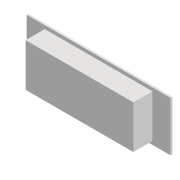
# Autodesk Inventor part: 00_FluidicChip_Vittorio
Saved by Autodesk Inventor 2022 (Build 260153000, 153)
## iProperties
Created: 2021-12-01
Part Number: 00_FluidicChip_Vittorio
Material: Generisch
Document SubType Name: Modeling
Designer: diederichbenedict
Density: 1 g/cm^3
Appearance: Vorgabe
Author: diederichbenedict
Autodesk Inventor part; units mm, degrees
ref_plane "YZ Plane" through (0, 0, 0) normal (1, 0, 0) x (0, 1, 0)
ref_plane "XZ Plane" through (0, 0, 0) normal (0, 1, 0) x (-1, 0, 0)
ref_plane "XY Plane" through (0, 0, 0) normal (0, 0, 1) x (1, 0, 0)
sketch "Skizze1" plane through (0, 0, 0) normal (0, 0, 1) x (1, 0, 0)
  line L0 (37.5, -13) -> (-37.5, -13)
  line L1 (-37.5, -13) -> (-37.5, 13)
  line L2 (-37.5, 13) -> (37.5, 13)
  line L3 (37.5, 13) -> (37.5, -13)
  line L4 (37.5, -13) -> (-37.5, 13) construction
  line L5 (-37.5, -13) -> (37.5, 13) construction
  point P0 (0, 0)
  dimension "d0" = 75
  dimension "d1" = 26
  constraints: 12 end point, 2 midpoint, 2 parallel, 1 horizontal, 1 perpendicular
  measures "d0" distance of L1.end L2.end
  measures "d1" distance of L0.end L1.end
extrude "Extrusion1" add sketch "Skizze1" along normal blind 1
sketch "Skizze2" plane through (0, 0, 1) normal (0, 0, 1) x (1, 0, 0)
  line L0 (37.5, 13) -> (-37.5, 13) projected
  line L1 (-37.5, 13) -> (-37.5, -13) projected
  line L2 (-37.5, -13) -> (37.5, -13) projected
  line L3 (37.5, -13) -> (37.5, 13) projected
  line L4 (28.1272, -11.233) -> (-28.1272, -11.233)
  line L5 (-28.1272, -11.233) -> (-28.1272, 11.233)
  line L6 (-28.1272, 11.233) -> (28.1272, 11.233)
  line L7 (28.1272, 11.233) -> (28.1272, -11.233)
  line L8 (28.1272, -11.233) -> (-28.1272, 11.233) construction
  line L9 (-28.1272, -11.233) -> (28.1272, 11.233) construction
  point P0 (0, 0)
  constraints: 12 end point, 2 midpoint, 2 parallel, 1 horizontal, 1 perpendicular
extrude "Extrusion2" add sketch "Skizze2" along normal blind 10 contours L4 L5 L6 L7
ref_plane "Arbeitsebene1" through (-37.5, 0, 0) normal (0, -1, 0) x (1, 0, 0)
ref_plane "Arbeitsebene2" through (0, -13, 0) normal (1, 0, 0) x (0, 0, -1)
